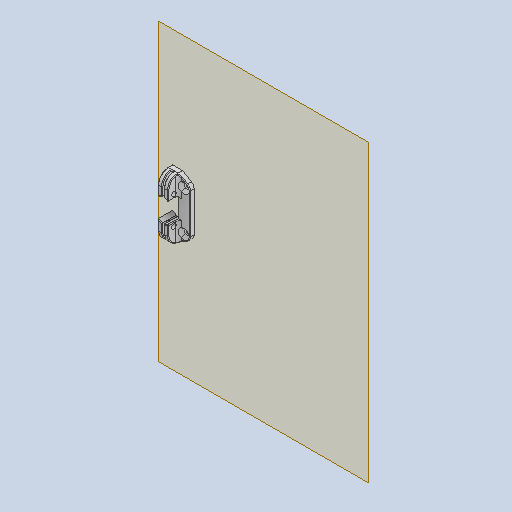
# Autodesk Inventor part: lazer_krepl
Saved by Autodesk Inventor 2022 (Build 260153000, 153)
## iProperties
Created: 2022-12-28
Part Number: lazer_krepl
Material: Типовые
Document SubType Name: Modeling
Designer: akapu
Density: 1 g/cm^3
Appearance: По умолчанию
Author: akapu
Autodesk Inventor part; units mm, degrees
ref_plane "YZ Plane" through (0, 0, 0) normal (1, 0, 0) x (0, 1, 0)
ref_plane "XZ Plane" through (0, 0, 0) normal (0, 1, 0) x (-1, 0, 0)
ref_plane "XY Plane" through (0, 0, 0) normal (0, 0, 1) x (1, 0, 0)
sketch "Эскиз1" plane through (0, 0, 0) normal (0, 0, 1) x (1, 0, 0)
  line L0 (-23.978, 76.75) -> (-44, 76.75) projected
  line L1 (-44, 76.75) -> (-44, 88.75) projected
  line L2 (-44, 88.75) -> (-23.978, 88.75) projected
  line L3 (-23.978, 88.75) -> (-23.978, 76.75) projected
  circle A0 centre (16.23, 81.75) radius 1.6 projected
  line L4 (23.978, 88.75) -> (44, 88.75) projected
  line L5 (44, 88.75) -> (44, 76.75) projected
  line L6 (44, 76.75) -> (23.978, 76.75) projected
  line L7 (23.978, 76.75) -> (23.978, 88.75) projected
  circle A1 centre (-16.23, 81.75) radius 1.6 projected
  circle A2 centre (-18, -71.75) radius 1.5 projected
  circle A3 centre (-18, 71.75) radius 1.5 projected
  circle A4 centre (48, -85.75) radius 1.5 projected
  circle A5 centre (-48, -85.75) radius 1.5 projected
  circle A6 centre (48, 71.75) radius 1.5 projected
  circle A7 centre (-48, 71.75) radius 1.5 projected
  circle A8 centre (18, -71.75) radius 1.5 projected
  circle A9 centre (-48, -71.75) radius 1.5 projected
  circle A10 centre (18, 71.75) radius 1.5 projected
  circle A11 centre (18, -85.75) radius 1.5 projected
  circle A12 centre (-18, -85.75) radius 1.5 projected
  circle A13 centre (48, 85.75) radius 1.5 projected
  circle A14 centre (-48, 85.75) radius 1.5 projected
  circle A15 centre (48, -71.75) radius 1.5 projected
  line L8 (-63, -85.75) -> (-63, 85.75) projected
  line L9 (-63, -85.75) -> (-66, -85.75) projected
  line L10 (-66, -92.75) -> (-66, -85.75) projected
  line L11 (66, -92.75) -> (-66, -92.75) projected
  line L12 (66, -85.75) -> (66, -92.75) projected
  line L13 (66, -85.75) -> (63, -85.75) projected
  line L14 (63, -85.75) -> (63, 85.75) projected
  line L15 (63, 85.75) -> (66, 85.75) projected
  line L16 (66, 92.75) -> (66, 85.75) projected
  line L17 (-66, 92.75) -> (66, 92.75) projected
  line L18 (-66, 85.75) -> (-66, 92.75) projected
  line L19 (-66, 85.75) -> (-63, 85.75) projected
  circle A16 centre (-42, 57.75) radius 1.6 projected
  circle A17 centre (56, 57.75) radius 1.6 projected
  circle A18 centre (42, -41.75) radius 1.6 projected
  circle A19 centre (-56, -57.75) radius 1.6 projected
  circle A20 centre (-56, -41.75) radius 1.6 projected
  circle A21 centre (42, -57.75) radius 1.6 projected
  circle A22 centre (42, 41.75) radius 1.6 projected
  circle A23 centre (-56, 41.75) radius 1.6 projected
  circle A24 centre (-56, 57.75) radius 1.6 projected
  circle A25 centre (42, 57.75) radius 1.6 projected
  circle A26 centre (56, -41.75) radius 1.6 projected
  circle A27 centre (-42, -41.75) radius 1.6 projected
  circle A28 centre (-42, -57.75) radius 1.6 projected
  circle A29 centre (56, -57.75) radius 1.6 projected
  circle A30 centre (56, 41.75) radius 1.6 projected
  circle A31 centre (-42, 41.75) radius 1.6 projected
  circle A32 centre (6.2, -33.75) radius 3 projected
  circle A33 centre (-6.2, 33.75) radius 3 projected
  circle A34 centre (-6.2, -33.75) radius 3 projected
  circle A35 centre (6.2, 33.75) radius 3 projected
  circle A36 centre (42.6, 16.75) radius 1.5 projected
  circle A37 centre (-42.6, 16.75) radius 1.5 projected
  circle A38 centre (42.6, -16.75) radius 1.5 projected
  circle A39 centre (-42.6, -16.75) radius 1.5 projected
  line L20 (-38, -8.35) -> (-41, -8.35) projected
  line L21 (-41, -8.35) -> (-41, 8.35) projected
  line L22 (-41, 8.35) -> (-38, 8.35) projected
  line L23 (-38, 8.35) -> (-38, 18.35) projected
  line L24 (-38, 18.35) -> (38, 18.35) projected
  line L25 (38, 18.35) -> (38, 8.35) projected
  line L26 (38, 8.35) -> (41, 8.35) projected
  line L27 (41, 8.35) -> (41, -8.35) projected
  line L28 (41, -8.35) -> (38, -8.35) projected
  line L29 (38, -8.35) -> (38, -18.35) projected
  line L30 (38, -18.35) -> (-38, -18.35) projected
  line L31 (-38, -18.35) -> (-38, -8.35) projected
  line L32 (-63, 0) -> (-63, 9.75)
  line L33 (-63, 9.75) -> (-60, 9.75)
  line L34 (-63, 9.75) -> (-63, -9.75)
  line L35 (-63, -9.75) -> (-60, -9.75)
  line L36 (-60, 9.75) -> (-58.8, 9.75)
  line L37 (-58.8, 9.75) -> (-55.8, 9.75)
  line L38 (-60, 9.75) -> (-60, 8.25)
  line L39 (-60, 8.25) -> (-60, 7.95)
  line L40 (-63, 9.75) -> (-63, 6.75)
  line L41 (-63, 6.75) -> (-60, 7.95)
  line L42 (-58.8, 9.75) -> (-58.8, 7.95)
  line L43 (-58.8, 7.95) -> (-55.8, 6.75)
  line L44 (-55.8, 6.75) -> (-55.8, 12.75)
  line L45 (-58.8, 9.75) -> (-58.8, 11.55)
  line L46 (-60, 9.75) -> (-60, 11.55)
  line L47 (-63, 9.75) -> (-63, 12.75)
  line L48 (-63, 0) -> (-55.8, 0)
  line L49 (-60, -9.75) -> (-60, -11.25)
  line L50 (-60, -11.25) -> (-60, -11.55)
  line L51 (-58.8, -9.75) -> (-58.8, -11.55)
  line L52 (-55.8, -12.75) -> (-55.8, -6.75)
  line L53 (-58.8, -9.75) -> (-58.8, -7.95)
  line L54 (-58.8, -7.95) -> (-55.8, -6.75)
  line L55 (-60, -9.75) -> (-60, -7.95)
  line L56 (-60, -7.95) -> (-63, -6.75)
  line L57 (-55.8, -12.75) -> (-55.8, -20.75)
  line L58 (-55.8, -20.75) -> (-63, -20.75)
  line L59 (-55.8, 12.75) -> (-55.8, 20.75)
  line L60 (-55.8, 20.75) -> (-63, 20.75)
  line L61 (-58.8, 11.55) -> (-58.8, 20.75)
  line L62 (-60, 11.55) -> (-60, 20.75)
  line L63 (-58.8, -11.55) -> (-58.8, -20.75)
  line L64 (-60, -11.55) -> (-60, -20.75)
  line L65 (-55.8, 12.75) -> (-55.8, 13.75)
  line L66 (-55.8, 13.75) -> (-51.8, 13.75)
  line L67 (-55.8, -12.75) -> (-55.8, -13.75)
  line L68 (-55.8, -13.75) -> (-51.8, -13.75)
  circle A40 centre (-51.8, 13.75) radius 1.6
  circle A41 centre (-51.8, -13.75) radius 1.6
  circle A42 centre (-51.8, -13.75) radius 4
  circle A43 centre (-51.8, 13.75) radius 4
  line L69 (-55.8, 20.75) -> (-49.7692, 17.1962)
  line L70 (-55.8, -20.75) -> (-49.7692, -17.1962)
  line L71 (-47.8, -13.75) -> (-47.8, 13.75)
  circle A44 centre (51.8, -13.75) radius 1.5 projected
  circle A45 centre (-51.8, -13.75) radius 1.5 projected
  circle A46 centre (51.8, 13.75) radius 1.5 projected
  circle A47 centre (-51.8, 13.75) radius 1.5 projected
  point P0 (0, 0)
  dimension "d0" = 9.75
  dimension "d1" = 3
  dimension "d2" = 19.5
  dimension "d3" = 3
  dimension "d4" = 1.2
  dimension "d5" = 3
  dimension "d6" = 1.5
  dimension "d7" = 0.3
  dimension "d8" = 3
  dimension "d9" = 6
  dimension "d10" = 1.8
  dimension "d11" = 1.2
  dimension "d12" = 1.5
  dimension "d14" = 6
  dimension "d15" = 1.8
  dimension "d16" = 8
  dimension "d17" = 8
  dimension "d18" = 1
  dimension "d19" = 4
  dimension "d20" = 1
  dimension "d21" = 3.2
  dimension "d22" = 3.2
  constraints: 80 end point, 18 point on line, 9 vertical, 8 perpendicular, 6 point on circle, 4 centre point, 4 coincident, 3 tangent, 2 horizontal, 2 parallel, 1 collinear, 1 midpoint
  measures "d0" distance of L32.start L32.end
  measures "d1" distance of L32.end L33.end
  measures "d2" distance of L32.end L34.end
  measures "d3" distance of L34.end L35.end
  measures "d4" distance of L33.end L36.end
  measures "d5" distance of L36.end L37.end
  measures "d6" distance of L33.end L38.end
  measures "d7" distance of L38.end L39.end
  measures "d8" distance of L32.end L40.end
  measures "d9" distance of L43.end L44.end
  measures "d10" distance of L36.end L45.end
  measures "d11" distance of L49.start L51.start
  measures "d12" distance of L49.start L50.start
  measures "d14" distance of L52.start L52.end
  measures "d15" distance of L51.start L53.end
  measures "d16" distance of L52.start L57.end
  measures "d17" distance of L44.end L59.end
  measures "d18" distance of L44.end L65.end
  measures "d19" distance of L65.end L66.end
  measures "d20" distance of L52.start L67.end
  measures "d21" diameter of A40
  measures "d22" diameter of A41
extrude "Выдавливание1" add sketch "Эскиз1" along normal blind 10 contours L8 L35 L49 L50 L64 L58 | L8 L56 L55 L35 | L63 L51 L53 L54 L52 L57 L58 | L8 L33 L38 L39 L41 | L8 L60 L62 L46 L33 | L45 L61 L60 L59 L44 L37 | L37 L44 L43 L42
ref_plane "РабПлоскость1" through (0, 0, 0) normal (0, 0, 1) x (1, 0, 0)
sketch "Эскиз2" plane through (0, 0, 0) normal (0, 0, 1) x (1, 0, 0)
  line L0 (-60, 20.75) -> (-63, 20.75) projected
  line L1 (-55.8, -20.75) -> (-55.8, -6.75) projected
  line L2 (-63, 20.75) -> (-55.8, 20.75)
  line L3 (-55.8, 20.75) -> (-55.8, -20.75)
  line L4 (-55.8, -20.75) -> (-63, -20.75)
  line L5 (-63, -20.75) -> (-63, 20.75)
  line L6 (-55.8, 20.75) -> (-58.8, 20.75) projected
  line L7 (-55.8, 20.75) -> (-49.7692, 17.1962)
  circle A0 centre (-51.8, 13.75) radius 4 projected
  line L8 (-55.8, -20.75) -> (-49.7692, -17.1962)
  circle A1 centre (-51.8, -13.75) radius 4 projected
  circle A2 centre (-51.8, -13.75) radius 4 projected
  circle A3 centre (-51.8, -13.75) radius 1.6 projected
  circle A4 centre (-51.8, 13.75) radius 4 projected
  circle A5 centre (-51.8, 13.75) radius 1.6 projected
  line L9 (-47.8, -13.75) -> (-47.8, 13.75)
  line L10 (-63, 0) -> (-55.8, 0)
  line L11 (-59.4, 0) -> (-59.4, 9.75)
  line L12 (-59.4, 9.75) -> (-59.4, 11.55)
  line L13 (-59.4, 11.55) -> (-60, 11.55)
  line L14 (-60, 7.95) -> (-60, 20.75) projected
  line L15 (-58.8, 11.55) -> (-59.4, 11.55)
  line L16 (-59.4, -11.55) -> (-60, -11.55)
  line L17 (-58.8, -11.55) -> (-59.4, -11.55)
  line L18 (-60, -20.75) -> (-60, -7.95) projected
  line L19 (-60, -20.75) -> (-58.8, -20.75)
  line L20 (-58.8, -20.75) -> (-58.8, -11.55)
  line L21 (-58.8, -11.55) -> (-60, -11.55)
  line L22 (-60, -11.55) -> (-60, -20.75)
  line L23 (-60, 11.55) -> (-58.8, 11.55)
  line L24 (-58.8, 11.55) -> (-58.8, 20.75)
  line L25 (-58.8, 20.75) -> (-60, 20.75)
  line L26 (-60, 20.75) -> (-60, 11.55)
  point P0 (0, 0)
  point P1 (-55.8, -13.75)
  point P2 (-55.8, 13.75)
  point P3 (-55.8, -13.75)
  point P4 (-55.8, 13.75)
  point P5 (-47.8, 13.75)
  dimension "d25" = 9.75
  dimension "d26" = 1.8
  constraints: 44 end point, 7 equal length, 4 perpendicular, 4 point on circle, 4 point on line, 3 horizontal, 3 midpoint, 3 symmetric about line, 3 tangent, 1 vertical
  measures "d25" distance of L11.start L11.end
  measures "d26" distance of L11.end L12.end
extrude "Выдавливание2" add sketch "Эскиз2" along normal blind 3 contours L2 L24 L15 L13 L14 | L7 A0 L3 | A0 L9 A1 L1 L3 | A0 | L18 L16 L17 L20 L4 | A1 | L1 A1 L8
fillet "Сопряжение1" radius 2 2 edges at (-55.8, 13.75, 3) (-55.8, -13.75, 3)
chamfer "Фаска1" distance 2 angle 45 2 edges at (-53.4, -13.75, 3) (-53.4, 13.75, 3)
fillet "Сопряжение2" radius 7 4 edges at (-57.3, -20.75, 10) (-61.5, -20.75, 10) (-57.3, 20.75, 10) (-61.5, 20.75, 10)
fillet "Сопряжение3" radius 0.5 37 edges at (-55.8, 0, 3) (-55.2142, 6.5157, 3.5858) (-55.8, 6.75, 7.5) (-55.2142, -6.5157, 3.5858) (-55.8, -6.75, 7.5) (-57.3, -7.35, 10) (-61.5, -7.35, 10) (-57.3, 7.35, 10) (-61.5, 7.35, 10) (-63, 6.75, 5) (-63, 18.6997, 7.9497) (-63, 20.75, 1.5) (-63, 10.25, 10) (-55.8, 17.9333, 8.6125) (-55.7562, 20.5685, 4.5838) (-55.8, 10.25, 10) (-55.8, -10.25, 10) (-55.7562, -20.5685, 4.5838) (-55.8, -17.9333, 8.6125) (-63, -20.75, 1.5) (-63, -10.25, 10) (-63, -18.6997, 7.9497) (-51.7846, -18.3838, 3) (-48.327, -15.7346, 3) (-47.8, 0, 3) (-48.327, 15.7346, 3) (-51.7846, 18.3838, 3) (-54.8899, 20.2137, 3.3231) (-54.8899, -20.2137, 3.3231) (-58.8, -10.85, 10) (-58.8, -18.6997, 7.9497) (-60, -10.85, 10) (-60, -18.6997, 7.9497) (-60, 18.6997, 7.9497) (-60, 10.85, 10) (-58.8, 18.6997, 7.9497) (-58.8, 10.85, 10)
sketch "Эскиз3" plane through (-63, 7.4885, 0) normal (-1, 0, 0) x (0, 0, 1)
  line L0 (0, -7.4885) -> (6, -7.4885)
  line L1 (0, -7.4885) -> (6, -7.4885) construction
  line L2 (6, -7.4885) -> (6, 2.2615)
  line L3 (6, 2.2615) -> (6, -17.2385)
  circle A0 centre (6, 2.2615) radius 1.6
  circle A1 centre (6, -17.2385) radius 1.6
  dimension "d35" = 6
  dimension "d36" = 0
  dimension "d37" = 9.75
  dimension "d38" = 19.5
  dimension "d39" = 3.2
  dimension "d40" = 3.2
  constraints: 8 end point, 2 centre point, 2 coincident, 2 horizontal, 1 collinear, 1 perpendicular, 1 point on line
  measures "d35" distance of L0.start L0.end
  measures "d36" distance between parallel lines of L0 L1
  measures "d37" distance of L0.end L2.end
  measures "d38" distance of L2.end L3.end
  measures "d39" diameter of A0
  measures "d40" diameter of A1
extrude "Выдавливание3" cut sketch "Эскиз3" against normal up to surface (7.2 mm away)
